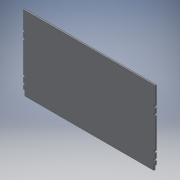
# Autodesk Inventor part: Print Platform
Saved by Autodesk Inventor 2019 (Build 230136000, 136)
## iProperties
Created: 2020-03-07
Part Number: Print Platform
Material: Generic
Document SubType Name: Modeling
Designer: Vijay
Density: 1 g/cm^3
Appearance: Default
Author: Vijay
Autodesk Inventor part; units mm, degrees
ref_plane "YZ Plane" through (0, 0, 0) normal (1, 0, 0) x (0, 1, 0)
ref_plane "XZ Plane" through (0, 0, 0) normal (0, 1, 0) x (-1, 0, 0)
ref_plane "XY Plane" through (0, 0, 0) normal (0, 0, 1) x (1, 0, 0)
sketch "Sketch1" plane through (0, 0, 0) normal (0, 0, 1) x (1, 0, 0)
  line L0 (200, -115) -> (-200, -115)
  line L1 (-200, -115) -> (-200, 115)
  line L2 (-200, 115) -> (200, 115)
  line L3 (200, 115) -> (200, -115)
  line L4 (200, -115) -> (-200, 115) construction
  line L5 (-200, -115) -> (200, 115) construction
  point P0 (0, 0)
  dimension "d0" = 400
  dimension "d1" = 230
  constraints: 12 end point, 2 midpoint, 2 parallel, 1 horizontal, 1 perpendicular
  measures "d0" distance of L1.end L2.end
  measures "d1" distance of L2.end L0.start
extrude "Extrusion1" add sketch "Sketch1" along normal blind 4
sketch "Sketch4" plane through (0, 0, 4) normal (0, 0, 1) x (1, 0, 0)
  line L0 (200, -99) -> (200, -88) projected
  line L1 (204, -99) -> (200, -99) projected
  line L2 (204, -88) -> (204, -99) projected
  line L3 (204, -88) -> (200, -88) projected
  line L4 (-204, -99) -> (-204, -88) projected
  line L5 (-200, -99) -> (-204, -99) projected
  line L6 (-200, -88) -> (-200, -99) projected
  line L7 (-200, -88) -> (-204, -88) projected
  line L8 (200, 115) -> (-200, 115) projected
  line L9 (204, -88) -> (-204, -88)
  line L10 (-204, -88) -> (-204, 115)
  line L11 (-204, 115) -> (204, 115)
  line L12 (204, 115) -> (204, -88)
  point P0 (0, 0)
  constraints: 8 end point, 2 parallel, 1 horizontal, 1 perpendicular
extrude "Extrusion4" add sketch "Sketch4" against normal up to surface (4 mm away)
sketch "Sketch5" plane through (0, 0, 4) normal (0, 0, 1) x (1, 0, 0)
  line L0 (200, -82) -> (200, -88) construction
  line L1 (204, -88) -> (200, -88) construction
  line L2 (204, -88) -> (204, -82) construction
  line L3 (204, -82) -> (200, -82) construction
  line L4 (200, -60.8) -> (200, -66.8) construction
  line L5 (204, -66.8) -> (200, -66.8) construction
  line L6 (204, -66.8) -> (204, -60.8) construction
  line L7 (204, -60.8) -> (200, -60.8) construction
  line L8 (200, 60.1516) -> (200, 54.1516) construction
  line L9 (204, 54.1516) -> (200, 54.1516) construction
  line L10 (204, 54.1516) -> (204, 60.1516) construction
  line L11 (204, 60.1516) -> (200, 60.1516) construction
  line L12 (200, 38.9517) -> (200, 32.9516) construction
  line L13 (204, 32.9516) -> (200, 32.9516) construction
  line L14 (204, 32.9516) -> (204, 38.9517) construction
  line L15 (204, 38.9517) -> (200, 38.9517) construction
  line L16 (-204, -82) -> (-204, -88) construction
  line L17 (-200, -88) -> (-204, -88) construction
  line L18 (-200, -88) -> (-200, -82) construction
  line L19 (-200, -82) -> (-204, -82) construction
  line L20 (-204, 60.1516) -> (-204, 54.1516) construction
  line L21 (-200, 54.1516) -> (-204, 54.1516) construction
  line L22 (-200, 54.1516) -> (-200, 60.1516) construction
  line L23 (-200, 60.1516) -> (-204, 60.1516) construction
  line L24 (-204, 38.9517) -> (-204, 32.9516) construction
  line L25 (-200, 32.9516) -> (-204, 32.9516) construction
  line L26 (-200, 32.9516) -> (-200, 38.9517) construction
  line L27 (-200, 38.9517) -> (-204, 38.9517) construction
  line L28 (-204, -60.8) -> (-204, -66.8) construction
  line L29 (-200, -66.8) -> (-204, -66.8) construction
  line L30 (-200, -66.8) -> (-200, -60.8) construction
  line L31 (-200, -60.8) -> (-204, -60.8) construction
  line L32 (200, -75.9) -> (200, -72.9) construction
  line L33 (204, -75.9) -> (200, -75.9) construction
  line L34 (204, -72.9) -> (204, -75.9) construction
  line L35 (204, -72.9) -> (200, -72.9) construction
  line L36 (200, 45.0517) -> (200, 48.0516) construction
  line L37 (204, 45.0517) -> (200, 45.0517) construction
  line L38 (204, 48.0516) -> (204, 45.0517) construction
  line L39 (204, 48.0516) -> (200, 48.0516) construction
  line L40 (-204, -75.9) -> (-204, -72.9) construction
  line L41 (-200, -75.9) -> (-204, -75.9) construction
  line L42 (-200, -72.9) -> (-200, -75.9) construction
  line L43 (-200, -72.9) -> (-204, -72.9) construction
  line L44 (-204, 45.0517) -> (-204, 48.0516) construction
  line L45 (-200, 45.0517) -> (-204, 45.0517) construction
  line L46 (-200, 48.0516) -> (-200, 45.0517) construction
  line L47 (-200, 48.0516) -> (-204, 48.0516) construction
  circle A0 centre (202, -74.4) radius 1.5
  circle A1 centre (-202, -74.4) radius 1.5
  circle A2 centre (-202, 46.5516) radius 1.5
  circle A3 centre (202, 46.5516) radius 1.5
  line L48 (199.9, -88.1) -> (199.9, -81.9)
  line L49 (199.9, -81.9) -> (204.1, -81.9)
  line L50 (204.1, -81.9) -> (204.1, -88.1)
  line L51 (204.1, -88.1) -> (199.9, -88.1)
  line L52 (199.9, -66.9) -> (199.9, -60.7)
  line L53 (199.9, -60.7) -> (204.1, -60.7)
  line L54 (204.1, -60.7) -> (204.1, -66.9)
  line L55 (204.1, -66.9) -> (199.9, -66.9)
  line L56 (199.9, 39.0517) -> (199.9, 32.8516)
  line L57 (199.9, 32.8516) -> (204.1, 32.8516)
  line L58 (204.1, 32.8516) -> (204.1, 39.0517)
  line L59 (204.1, 39.0517) -> (199.9, 39.0517)
  line L60 (199.9, 54.0516) -> (199.9, 60.2516)
  line L61 (199.9, 60.2516) -> (204.1, 60.2516)
  line L62 (204.1, 60.2516) -> (204.1, 54.0516)
  line L63 (204.1, 54.0516) -> (199.9, 54.0516)
  line L64 (-204.1, -81.9) -> (-204.1, -88.1)
  line L65 (-204.1, -88.1) -> (-199.9, -88.1)
  line L66 (-199.9, -88.1) -> (-199.9, -81.9)
  line L67 (-199.9, -81.9) -> (-204.1, -81.9)
  line L68 (-204.1, -66.9) -> (-204.1, -60.7)
  line L69 (-204.1, -60.7) -> (-199.9, -60.7)
  line L70 (-199.9, -60.7) -> (-199.9, -66.9)
  line L71 (-199.9, -66.9) -> (-204.1, -66.9)
  line L72 (-204.1, 32.8516) -> (-204.1, 39.0517)
  line L73 (-204.1, 39.0517) -> (-199.9, 39.0517)
  line L74 (-199.9, 39.0517) -> (-199.9, 32.8516)
  line L75 (-199.9, 32.8516) -> (-204.1, 32.8516)
  line L76 (-204.1, 60.2516) -> (-204.1, 54.0516)
  line L77 (-204.1, 54.0516) -> (-199.9, 54.0516)
  line L78 (-199.9, 54.0516) -> (-199.9, 60.2516)
  line L79 (-199.9, 60.2516) -> (-204.1, 60.2516)
  point P0 (0, 0)
  dimension "d52" = 3
  dimension "d53" = 3
  dimension "d54" = 3
  dimension "d55" = 3
  dimension "d58" = 0.1
  dimension "d59" = 0.1
  dimension "d60" = 0.1
  dimension "d61" = 0.1
  dimension "d62" = 0.1
  dimension "d63" = 0.1
  dimension "d64" = 0.1
  dimension "d65" = 0.1
  constraints: 64 end point, 4 centre point, 24 other
  measures "d52" diameter of A0
  measures "d53" diameter of A1
  measures "d54" diameter of A2
  measures "d55" diameter of A3
  measures "d58" distance between parallel lines of L0 L48
  measures "d59" distance between parallel lines of L5 L55
  measures "d60" distance between parallel lines of L15 L59
  measures "d61" distance between parallel lines of L9 L63
  measures "d62" distance between parallel lines of L19 L67
  measures "d63" distance between parallel lines of L29 L71
  measures "d64" distance between parallel lines of L25 L75
  measures "d65" distance between parallel lines of L23 L79
extrude "Extrusion5" cut sketch "Sketch5" against normal blind 10
body "Solid1"
